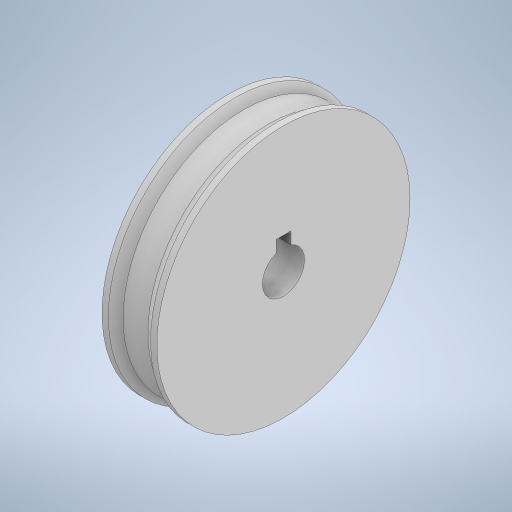
# Autodesk Inventor part: POLEA
Saved by Autodesk Inventor 2024 (Build 280153000, 153)
## iProperties
Created: 2024-03-01
Part Number: POLEA
Material: Generic
Document SubType Name: Modeling
Designer: augus
Density: 1 g/cm^3
Appearance: Default
Author: augus
Autodesk Inventor part; units mm, degrees
ref_plane "YZ Plane" through (0, 0, 0) normal (1, 0, 0) x (0, 1, 0)
ref_plane "XZ Plane" through (0, 0, 0) normal (0, 1, 0) x (-1, 0, 0)
ref_plane "XY Plane" through (0, 0, 0) normal (0, 0, 1) x (1, 0, 0)
sketch "Sketch1" plane through (0, 0, 0) normal (0, 0, 1) x (1, 0, 0)
  line L0 (0, 0) -> (0, 50)
  line L1 (20, 50) -> (20, 0)
  line L2 (20, 0) -> (0, 0)
  line L3 (0, -10) -> (-48.3632, -10)
  line L4 (0, 50) -> (4.0958, 47.1321)
  line L5 (20, 50) -> (15.9042, 47.1321)
  line L6 (4.0958, 47.1321) -> (15.9042, 47.1321)
  dimension "d3" = 10
  constraints: 14 end point, 1 horizontal, 1 point on line, 1 vertical
  measures "d3" distance of L0.start L3.start
revolve "Revolution1" add sketch "Sketch1" angle 360 about axis through (0, -10, 0) along (-1, 0, 0)
thicken "Thicken1" operation add thickness 3 both sides no extend neighbours no toward (-1, 0, 0) faces at (0, -50.5351, 14.7961)
thicken "Thicken2" operation add thickness 3 both sides no extend neighbours no toward (1, 0, 0) faces at (20, -50.5351, -14.7961)
sketch "Sketch2" plane through (-3, -10, 0) normal (-1, 0, 0) x (0, 0, 1)
  line L0 (-3.5, 5) -> (3.5, 5)
  line L1 (3.5, 5) -> (3.5, 15)
  line L2 (3.5, 15) -> (-3.5, 15)
  line L3 (-3.5, 15) -> (-3.5, 5)
  line L4 (-3.5, 5) -> (3.5, 15) construction
  line L5 (3.5, 5) -> (-3.5, 15) construction
  point P0 (0, 10)
  dimension "d11" = 7
  dimension "d12" = 10
  constraints: 12 end point, 2 midpoint, 2 parallel, 1 horizontal, 1 perpendicular
  measures "d11" distance of L2.end L1.end
  measures "d12" distance of L1.end L0.end
extrude "Extrusion1" cut sketch "Sketch2" against normal through all
